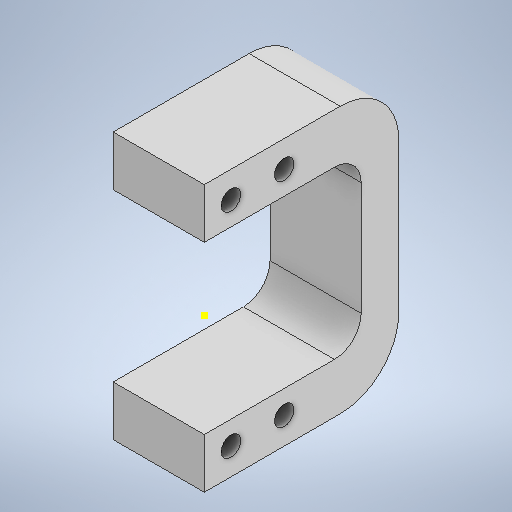
# Autodesk Inventor part: Front_support
Saved by Autodesk Inventor 2025.1 (Build 291241020, 241B)
## iProperties
Created: 2024-10-03
Part Number: Front_support
Material: Generic
Document SubType Name: Modeling
Designer: AtuStem
Density: 1 g/cm^3
Appearance: Default
Author: AtuStem
Autodesk Inventor part; units mm, degrees
ref_plane "YZ Plane" through (0, 0, 0) normal (1, 0, 0) x (0, 1, 0)
ref_plane "XZ Plane" through (0, 0, 0) normal (0, 1, 0) x (-1, 0, 0)
ref_plane "XY Plane" through (0, 0, 0) normal (0, 0, 1) x (1, 0, 0)
sketch "Sketch4" plane through (0, 0, 0) normal (0, 0, 1) x (1, 0, 0)
  line L0 (10.9923, 14.2423) -> (-9.6452, 14.2423)
  line L1 (11.786, 15.036) -> (11.786, 25.9263)
  line L2 (13.3735, 26.9423) -> (11.786, 26.9423)
  line L3 (-10.439, 15.036) -> (-10.439, 25.9263)
  line L4 (-10.439, 26.9423) -> (-12.0265, 26.9423)
  arc A0 (-10.439, 15.036) -> (-9.6452, 14.2423) centre (-9.6452, 15.036) ccw
  arc A1 (10.9923, 14.2423) -> (11.786, 15.036) centre (10.9923, 15.036) ccw
  arc A2 (11.786, -24.6515) -> (10.9923, -23.8577) centre (10.9923, -24.6515) ccw
  line L5 (-9.6452, -23.8577) -> (10.9923, -23.8577)
  arc A3 (-9.6452, -23.8577) -> (-10.439, -24.6515) centre (-9.6452, -24.6515) ccw
  line L6 (-10.439, -24.6515) -> (-10.439, -36.5577)
  line L7 (11.786, -24.6515) -> (11.786, -36.5577)
  line L8 (11.786, 26.9423) -> (11.786, 25.9263)
  line L9 (-10.439, 26.9423) -> (-10.439, 25.9263)
  line L10 (11.786, -24.6515) -> (-10.439, -24.6515)
  line L11 (11.786, 15.036) -> (-10.439, 15.036)
  line L12 (11.786, 26.9423) -> (11.532, 26.9423)
  line L13 (11.532, 26.9423) -> (11.532, 15.036)
  line L14 (-10.439, 26.9423) -> (-10.185, 26.9423)
  line L15 (-10.185, 26.9423) -> (-10.185, 15.036)
  line L16 (11.532, 26.9423) -> (-10.185, 26.9423)
  line L17 (11.786, -24.6515) -> (11.532, -24.6515)
  line L18 (11.532, -24.6515) -> (11.532, -36.5577)
  line L19 (11.532, -36.5577) -> (11.786, -36.5577)
  line L20 (11.786, -36.5577) -> (11.786, -24.6515)
  line L21 (-10.439, -24.6515) -> (-10.185, -24.6515)
  line L22 (-10.185, -24.6515) -> (-10.185, -36.5577)
  line L23 (-10.185, -36.5577) -> (-10.439, -36.5577)
  line L24 (-10.439, -36.5577) -> (-10.439, -24.6515)
  line L25 (11.532, -36.5577) -> (-10.439, -36.5577)
  line L26 (0, 14.2423) -> (0, -23.8577)
  point P0 (0, 0)
  dimension "d5" = 22.225
  dimension "d6" = 0.254
  dimension "d7" = 0.254
  dimension "d14" = 38.1
  constraints: 54 end point, 8 perpendicular, 8 point on circle, 5 parallel, 4 centre point, 4 horizontal, 4 point on line, 1 collinear, 1 vertical
  measures "d5" distance between parallel lines of L6 L7
  measures "d6" distance of L2.end L12.end
  measures "d7" distance of L4.start L14.end
  measures "d14" distance of L26.start L26.end
extrude "Extrusion2" add sketch "Sketch4" against normal blind 25.4 contours L11 L15 L16 L13 | L18 L25 L22 L10
sketch "Sketch5" plane through (11.532, -36.5577, 0) normal (1, 0, 0) x (0, 0, -1)
  point P0 (0, 36.5577)
sketch "Sketch6" plane through (11.532, -36.5577, 0) normal (1, 0, 0) x (0, 0, -1)
  line L0 (0, 51.5938) -> (0, 63.5) projected
  line L1 (0, 51.5938) -> (25.4, 51.5938) projected
  line L2 (25.4, 63.5) -> (25.4, 51.5938) projected
  line L3 (0, 63.5) -> (25.4, 63.5) projected
  line L4 (0, 0) -> (0, 11.9062) projected
  line L5 (0, 0) -> (25.4, 0) projected
  line L6 (25.4, 11.9062) -> (25.4, 0) projected
  line L7 (0, 11.9062) -> (25.4, 11.9062) projected
  line L8 (25.4, 63.5) -> (25.4, 57.15)
  line L9 (25.4, 57.15) -> (19.05, 57.15)
  line L10 (25.4, 0) -> (25.4, 6.35)
  line L11 (25.4, 6.35) -> (19.05, 6.35)
  line L12 (25.4, 62.484) -> (25.4, 51.5938)
  line L13 (37.3758, 42.3425) -> (37.3758, 45.2438)
  line L14 (37.3758, 63.5) -> (25.4, 63.5)
  line L15 (37.3758, 0) -> (25.4, 0)
  line L16 (25.4, 63.5) -> (37.3758, 63.5)
  line L17 (46.355, 51.9072) -> (46.355, 11.5928)
  line L18 (37.3758, 0) -> (25.4, 0)
  line L19 (25.4, 51.5938) -> (31.0258, 51.5938)
  line L20 (25.4, 11.9062) -> (31.0258, 11.9062)
  arc A0 (37.3758, 45.2438) -> (31.0258, 51.5938) centre (31.0258, 45.2438) ccw
  line L21 (46.355, 51.9072) -> (46.355, 50.8)
  arc A1 (46.355, 50.8) -> (37.3758, 63.5) centre (33.6671, 51.3536) ccw
  arc A2 (31.0258, 11.9062) -> (37.3758, 18.2562) centre (31.0258, 18.2562) ccw
  line L22 (46.355, 11.5928) -> (46.355, 12.7)
  arc A3 (37.3758, 0) -> (46.355, 12.7) centre (33.6671, 12.1464) ccw
  line L23 (37.3758, 42.3425) -> (37.3758, 18.2562)
  line L24 (25.4, 6.35) -> (19.05, 6.35)
  circle A4 centre (19.05, 57.15) radius 2.3241
  circle A5 centre (6.35, 57.15) radius 2.3241
  line L25 (25.4, 6.35) -> (19.05, 6.35)
  circle A6 centre (19.05, 6.35) radius 2.3241
  line L26 (19.05, 6.35) -> (6.35, 6.35)
  circle A7 centre (6.35, 6.35) radius 2.3241
  point P0 (0, 36.5577)
  dimension "d15" = 6.35
  dimension "d16" = 6.35
  dimension "d17" = 6.35
  dimension "d35" = 4.6482
  dimension "d36" = 4.6482
  dimension "d37" = 12.7
  dimension "d38" = 4.6482
  constraints: 38 end point, 10 point on circle, 9 perpendicular, 8 centre point, 4 point on line, 2 coincident, 2 horizontal, 1 vertical
  measures "d15" distance of L2.start L8.end
  measures "d16" distance of L8.end L9.end
  measures "d17" distance of L5.end L10.end
  measures "d35" diameter of A4
  measures "d36" diameter of A5
  measures "d37" distance of L26.start L26.end
  measures "d38" diameter of A7
extrude "Extrusion3" add sketch "Sketch6" against normal up to surface (21.717 mm away) contours L2 L14 A1 L17 A3 L15 L6 L20 A2 L23 L13 A0 L19
extrude "Extrusion4" cut sketch "Sketch6" along normal through all both and the other way through all contours A6 L26 L11 | L11 L26 A6 | A4 | A5 | A7
fillet "Fillet1" radius 13.97 2 edges at (0.6735, 26.9423, -37.3758) (0.6735, -36.5577, -37.3758)
fillet_without_effect "Fillet2"
body "Solid2"
